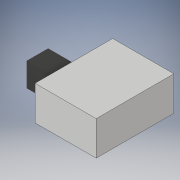
# Autodesk Inventor part: 103-5007-EV
Saved by Autodesk Inventor 2019.4 (Build 234330000, 330)
## iProperties
Created: 2020-02-03
Part Number: 103-5007-EV
Material: Generic
Document SubType Name: Modeling
Designer: Lars larsen
Density: 1 g/cm^3
Appearance: Default
Author: Lars larsen
Autodesk Inventor part; units mm, degrees
ref_plane "YZ Plane" through (0, 0, 0) normal (1, 0, 0) x (0, 1, 0)
ref_plane "XZ Plane" through (0, 0, 0) normal (0, 1, 0) x (-1, 0, 0)
ref_plane "XY Plane" through (0, 0, 0) normal (0, 0, 1) x (1, 0, 0)
sketch "Sketch1" plane through (0, 0, 0) normal (0, 1, 0) x (-1, 0, 0)
  line L0 (0, 0) -> (10, 0)
  line L1 (10, 0) -> (10, -12.7)
  line L2 (10, -12.7) -> (0, -12.7)
  line L3 (0, -12.7) -> (0, 0)
  dimension "d0" = 10
  dimension "d1" = 12.7
  constraints: 8 end point, 2 parallel, 1 horizontal, 1 perpendicular
  measures "d0" distance of L1.end L2.end
  measures "d1" distance between parallel lines of L0 L2
extrude "Extrusion1" add sketch "Sketch1" along normal blind 5.6
sketch "Sketch2" plane through (-10, 0, -12.7) normal (-1, 0, 0) x (0, 0, 1)
  line L0 (3.3, 4.8) -> (9.4, 4.8)
  line L1 (9.4, 4.8) -> (9.4, 0.8)
  line L2 (9.4, 0.8) -> (3.3, 0.8)
  line L3 (3.3, 0.8) -> (3.3, 4.8)
  line L4 (0, 0) -> (0, 5.6) projected
  point P0 (12.7, 0)
  point P1 (6.35, 4.8)
  point P2 (9.4, 2.8)
  dimension "d4" = 6.1
  dimension "d5" = 4
  dimension "d6" = 2.8
  dimension "d7" = 6.35
  constraints: 8 end point, 2 midpoint, 2 parallel, 1 horizontal, 1 perpendicular
  measures "d4" distance of L0.start L0.end
  measures "d5" distance of L0.end L1.end
  measures "d6" vertical distance of point (12.7, 0) point (9.4, 2.8)
  measures "d7" distance from line of L4 point (6.35, 4.8)
extrude "Extrusion2" cut sketch "Sketch2" against normal blind 1
sketch "Sketch3" plane through (-9, 0, -12.7) normal (-1, 0, 0) x (0, 0, 1)
  line L0 (5.8365, 4.7365) -> (9.3365, 4.7365)
  line L1 (9.3365, 4.7365) -> (9.3365, 0.8765)
  line L2 (9.3365, 0.8765) -> (5.8365, 0.8765)
  line L3 (5.8365, 0.8765) -> (5.8365, 4.7365)
  line L4 (9.4, 4.8) -> (9.4, 0.8) projected
  line L5 (3.3, 4.8) -> (9.4, 4.8) projected
  point P0 (12.7, 0)
  dimension "d10" = 3.5
  dimension "d11" = 3.86
  dimension "d12" = 0.0635
  dimension "d13" = 0.0635
  constraints: 8 end point, 2 parallel, 1 horizontal, 1 perpendicular
  measures "d10" distance between parallel lines of L1 L3
  measures "d11" distance of L0.end L1.end
  measures "d12" distance between parallel lines of L4 L1
  measures "d13" distance between parallel lines of L5 L0
extrude "Extrusion3" add sketch "Sketch3" along normal blind 5.72
body "Solid1"
